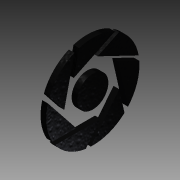
# Autodesk Inventor part: aperture
Saved by Autodesk Inventor 2015 (Build 190159000, 159)
## iProperties
Created: 2013-11-11
Part Number: aperture
Material: Generic
Document SubType Name: Modeling
Designer: Adam
Density: 1 g/cm^3
Appearance: Fine Textured - Black
Author: Adam
Autodesk Inventor part; units mm, degrees
ref_plane "YZ Plane" through (0, 0, 0) normal (1, 0, 0) x (0, 1, 0)
ref_plane "XZ Plane" through (0, 0, 0) normal (0, 1, 0) x (-1, 0, 0)
ref_plane "XY Plane" through (0, 0, 0) normal (0, 0, 1) x (1, 0, 0)
sketch "Sketch1" plane through (0, 0, 0) normal (1, 0, 0) x (0, 1, 0)
  circle A0 centre (0, 0) radius 42.0506 construction
  line L0 (0, 0) -> (25.4, 0) construction
  line L1 (25.4, 0) -> (15.8366, -19.8585) construction
  line L2 (15.8366, -19.8585) -> (-5.652, -24.7632) construction
  line L3 (-5.652, -24.7632) -> (-22.8846, -11.0206) construction
  line L4 (-22.8846, -11.0206) -> (-22.8846, 11.0206) construction
  line L5 (-22.8846, 11.0206) -> (-5.652, 24.7632) construction
  line L6 (-5.652, 24.7632) -> (15.8366, 19.8585) construction
  line L7 (15.8366, 19.8585) -> (25.4, 0) construction
  line L8 (-22.8846, -11.0206) -> (-41.8499, 4.1036) construction
  line L9 (-22.8846, 11.0206) -> (-22.8846, 35.2781) construction
  line L10 (-24.7896, -9.5015) -> (-24.7896, 33.9665) construction
  line L11 (-22.8846, -8.5841) -> (-41.573, 6.3194) construction
  line L12 (-24.7896, -7.0649) -> (-24.7896, 33.9665)
  line L13 (-24.7896, -7.0649) -> (-41.573, 6.3194)
  arc A1 (-24.7896, 33.9665) -> (-41.573, 6.3194) centre (0, 0) ccw
  line L14 (-9.9325, -23.7862) -> (-42.0122, 1.7965)
  line L15 (-9.9325, -23.7862) -> (-30.8611, -28.563)
  arc A2 (-42.0122, 1.7965) -> (-30.8611, -28.563) centre (0, 0) ccw
  line L16 (12.4039, -22.596) -> (-27.5987, -31.7263)
  line L17 (12.4039, -22.596) -> (3.0899, -41.9369)
  arc A3 (-27.5987, -31.7263) -> (3.0899, -41.9369) centre (0, 0) ccw
  line L18 (25.4, -4.3906) -> (7.5971, -41.3586)
  line L19 (25.4, -4.3906) -> (34.7141, -23.7315)
  arc A4 (7.5971, -41.3586) -> (34.7141, -23.7315) centre (0, 0) ccw
  line L20 (19.2693, 17.121) -> (37.0722, -19.847)
  line L21 (19.2693, 17.121) -> (40.1979, 12.3442)
  arc A5 (37.0722, -19.847) -> (40.1979, 12.3442) centre (0, 0) ccw
  line L22 (-1.3715, 25.7402) -> (38.6311, 16.6098)
  line L23 (-1.3715, 25.7402) -> (15.4119, 39.1245)
  arc A6 (38.6311, 16.6098) -> (15.4119, 39.1245) centre (0, 0) ccw
  line L24 (-20.9796, 14.9764) -> (11.1, 40.5591)
  line L25 (-20.9796, 14.9764) -> (-20.9796, 36.4432)
  arc A7 (11.1, 40.5591) -> (-20.9796, 36.4432) centre (0, 0) ccw
  dimension "d0" = 25.4
  dimension "d2" = 84.1011
  dimension "d3" = 1.905
  dimension "d4" = 1.905
  dimension "d7" = 360
  constraints: 52 end point, 18 point on circle, 8 centre point, 4 collinear, 4 point on line, 2 coincident, 2 parallel, 1 concentric, 1 horizontal, 65 other
  measures "d0" distance of L0.start L0.end
  measures "d2" diameter of A0
  measures "d3" distance between parallel lines of L10 L9
  measures "d4" distance between parallel lines of L8 L11
extrude "Extrusion1" add sketch "Sketch1" along normal blind 5.08
sketch "Sketch2" plane through (5.08, 0, 0) normal (1, 0, 0) x (0, 0, -1)
  circle A0 centre (0, 0) radius 14.0169
  circle A1 centre (0, 0) radius 42.0506 construction
  point P0 (19.847, 37.0722)
  dimension "d11" = 84.1011
  dimension "d12" = 28.0337
  constraints: 2 coincident, 1 centre point, 3 other
  measures "d12" diameter of A0
extrude "Extrusion2" add sketch "Sketch2" against normal up to surface (5.08 mm away)
equation "\"d2\" = 3.23607 * d0 + d3"
equation "\"d3\" = 0.075 * d0"
equation "\"d4\" = d3"
equation "\"d9\" = 0.2 * d0"
equation "\"d12\" = 0.333333 * d11"
body "Solid1"
